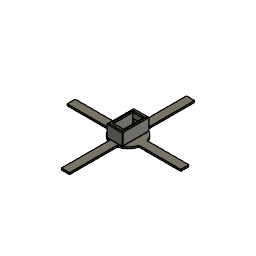
Davinki Base (Autodesk Fusion 360 design; units mm, degrees)
part number: 2026-08-29-10-07-06-773
Autodesk Fusion 360 part; units mm, degrees
note: some values were not read from the file. Set by a fixed rule: which sketch regions a step uses.
sketch "Sketch1" plane through (0, 0, 0) normal (0, 1, 0) x (1, 0, 0)
  line L0 (0, 0) -> (12.25, 0)
  line L1 (12.25, 0) -> (12.25, 23.5)
  line L2 (0, 0) -> (0, 23.5)
  line L3 (0, 23.5) -> (12.25, 23.5)
  line L4 (-3.4056, 0) -> (-3.4056, 27)
  line L5 (-3.4056, 27) -> (15.0988, 27)
  line L6 (15.0988, 27) -> (15.0988, -3.5)
  line L7 (15.0988, -3.5) -> (-3.4056, -3.5)
  line L8 (-3.4056, -3.5) -> (-3.4056, 27)
  line L9 (-3.4056, 27) -> (-3.4056, 28)
  line L10 (-3.4056, 28) -> (15.0988, 28)
  line L11 (15.0988, 28) -> (15.0988, 27)
  line L12 (-3.4056, -3.5) -> (-3.4056, -4.5)
  line L13 (-3.4056, -4.5) -> (15.1, -4.5)
  line L14 (15.1, -4.5) -> (15.0988, -3.5)
  line L15 (0, 23.5) -> (0, 0.25)
  line L16 (5.8472, -4.5) -> (5.8472, -29.5)
  line L17 (5.8472, -29.5) -> (10.8472, -29.5)
  line L18 (10.8472, -29.5) -> (0.8472, -29.5)
  line L19 (0.8472, -29.5) -> (0.8472, -4.5)
  line L20 (10.8472, -29.5) -> (10.8472, -4.5)
  line L21 (5.8466, 28) -> (5.8466, 53)
  line L22 (5.8466, 53) -> (10.8466, 53)
  line L23 (10.8466, 53) -> (0.8466, 53)
  line L24 (0.8466, 53) -> (0.8466, 28)
  line L25 (10.8466, 53) -> (10.8466, 28)
  line L26 (12.25, 11.75) -> (-3.4056, 11.75)
  line L27 (-3.4056, 11.75) -> (-28.4056, 11.75)
  line L28 (-28.4056, 11.75) -> (-28.4056, 6.75)
  line L29 (-28.4056, 6.75) -> (-28.4056, 16.75)
  line L30 (-28.4056, 16.75) -> (-3.4056, 16.7633)
  line L31 (-28.4056, 6.75) -> (-3.4056, 6.75)
  line L32 (15.0988, 11.75) -> (40.0988, 11.75)
  line L33 (40.0988, 11.75) -> (40.0988, 6.75)
  line L34 (40.0988, 6.75) -> (40.0988, 16.75)
  line L35 (40.0988, 16.75) -> (15.0988, 16.75)
  line L36 (40.0988, 6.75) -> (15.0988, 6.75)
  line L37 (-28.4056, 16.75) -> (-63.4056, 16.75)
  line L38 (-28.4056, 6.75) -> (-63.4056, 6.75)
  line L39 (-63.4056, 6.75) -> (-63.4056, 16.75)
  line L40 (40.0988, 16.75) -> (75.0988, 16.75)
  line L41 (75.0988, 16.75) -> (75.0988, 6.75)
  line L42 (75.0988, 6.75) -> (40.0988, 6.75)
  line L43 (10.8466, 53) -> (10.8466, 88)
  line L44 (0.8466, 53) -> (0.8466, 88)
  line L45 (0.8466, 88) -> (10.8466, 88)
  line L46 (10.8472, -29.5) -> (10.8472, -64.5)
  line L47 (10.8472, -64.5) -> (0.8466, -64.5)
  line L48 (0.8466, -64.5) -> (0.8472, -29.5)
  circle A0 centre (5.9954, 11.75) radius 18.8312
  dimension "d1" = 12.25
  dimension "d2" = 23.5
  dimension "d3" = 23.5
  dimension "d6" = 30.5
  dimension "d7" = 1
  dimension "d8" = 1
  dimension "d16" = 23.25
  dimension "d17" = 25
  dimension "d18" = 5
  dimension "d19" = 10
  dimension "d20" = 25
  dimension "d21" = 5
  dimension "d22" = 10
  dimension "d23" = 25
  dimension "d24" = 5
  dimension "d25" = 10
  dimension "d26" = 25
  dimension "d30" = 25
  dimension "d31" = 5
  dimension "d32" = 10
  dimension "d35" = 35
  dimension "d36" = 35
  dimension "d37" = 35
  dimension "d38" = 35
  dimension "d39" = 35
  dimension "d40" = 35
  constraint coincident L0.start L2.start
  constraint horizontal L0
  constraint perpendicular L0 L1
  constraint perpendicular L0 L2
  constraint horizontal L5
  constraint vertical L6
  constraint horizontal L7
  constraint vertical L8
  constraint perpendicular L5 L9
  constraint perpendicular L6 L10
  constraint perpendicular L5 L11
  constraint perpendicular L7 L12
  constraint perpendicular L8 L13
  constraint perpendicular L0 L15
  constraint midpoint L13 L16.start
  constraint perpendicular L13 L16
  constraint perpendicular L16 L17
  constraint perpendicular L16 L18
  constraint coincident L13 L19.end
  constraint perpendicular L13 L19
  constraint perpendicular L17 L20
  constraint midpoint L10 L21.start
  constraint perpendicular L10 L21
  constraint perpendicular L21 L22
  constraint perpendicular L21 L23
  constraint coincident L10 L24.end
  constraint perpendicular L10 L24
  constraint coincident L10 L25.end
  constraint perpendicular L10 L25
  constraint midpoint L1 L26.start
  constraint midpoint L8 L26.end
  constraint perpendicular L4 L26
  constraint perpendicular L8 L27
  constraint perpendicular L27 L28
  constraint perpendicular L27 L29
  constraint coincident L8 L30.end
  constraint perpendicular L8 L31
  constraint midpoint L6 L32.start
  constraint perpendicular L6 L32
  constraint perpendicular L32 L33
  constraint perpendicular L32 L34
  constraint coincident L6 L35.end
  constraint perpendicular L6 L35
  constraint coincident L6 L36.end
  constraint perpendicular L6 L36
  constraint perpendicular L29 L37
  constraint perpendicular L28 L38
  constraint perpendicular L34 L40
  constraint perpendicular L35 L41
  constraint perpendicular L34 L42
  constraint perpendicular L42 L43
  constraint perpendicular L23 L44
  constraint perpendicular L43 L45
  constraint perpendicular L18 L46
  constraint perpendicular L20 L47
  constraint coincident L26 A0.centre
  measures "d1" distance of L0.start L0.end
  measures "d2" distance of L0.end L1.end
  measures "d3" distance of L0.start L2.end
  measures "d6" distance of L4.end L7.end
  measures "d7" distance of L4.end L9.end
  measures "d8" distance of L7.end L12.end
  measures "d16" distance of L2.end L15.end
  measures "d17" distance of L16.start L16.end
  measures "d18" distance of L16.end L17.end
  measures "d19" distance of L17.end L18.end
  measures "d20" distance of L21.start L21.end
  measures "d21" distance of L21.end L22.end
  measures "d22" distance of L22.end L23.end
  measures "d23" distance of L26.end L27.end
  measures "d24" distance of L27.end L28.end
  measures "d25" distance of L28.end L29.end
  measures "d26" distance of L28.end L31.end
  measures "d30" distance of L32.start L32.end
  measures "d31" distance of L32.end L33.end
  measures "d32" distance of L33.end L34.end
  measures "d35" distance of L29.end L37.end
  measures "d36" distance of L28.end L38.end
  measures "d37" distance of L34.end L40.end
  measures "d38" distance of L22.end L43.end
  measures "d39" distance of L23.end L44.end
  measures "d40" distance of L17.end L46.end
extrude "Extrude1" add sketch "Sketch1" along normal blind 17.3 contours L4 L5 L6 L7 L8 | L7 L12 L13 L14 | L5 L9 L10 L11
sketch "Sketch2" plane through (0, 0, -28) normal (0, 0, -1) x (-1, 0, 0)
  line L0 (-15.0988, 0) -> (3.4056, 0)
  line L1 (3.4056, 0) -> (3.4056, 17.3)
  line L2 (3.4056, 17.3) -> (-15.0988, 17.3)
  line L3 (-15.0988, 17.3) -> (-15.0988, 0)
  line L4 (-11.5, 2) -> (-1.0253, 2)
  line L5 (-1.0253, 2) -> (-1.0253, 5)
  line L6 (-11.5, 5) -> (-11.5, 2)
  line L7 (-11.5, 5) -> (-11.5, 10)
  line L8 (-11.5, 10) -> (-1, 10)
  line L9 (-1, 10) -> (-1.0253, 5)
  dimension "d11" = 3
  constraint horizontal L4
  constraint vertical L5
  constraint vertical L6
  constraint perpendicular L7 L8
  measures "d11" distance of L4.start L6.start
extrude "Extrude2" cut sketch "Sketch2" against normal blind 16 contours L4 L5 L6 L7 L8 L9
fillet "Fillet1" radius 1 1 faces at (3.8981, 17.3, 3)
extrude "Extrude3" add sketch "Sketch1" along normal blind 2 contours L4 L8 L27 L31 A0 | L4 L8 L27 L30 A0 | L27 L28 L29 L31 A0 | L27 L29 L30 A0 | L16 L18 L19 A0 | L13 L16 L19 A0 | L6 L32 L36 A0 | L16 L17 L18 L20 A0 | L13 L16 L20 A0 | L6 L32 L35 A0 | L32 L33 L34 L36 A0 | L10 L21 L24 A0 | L21 L23 L24 A0 | L32 L34 L35 A0 | L10 L21 L25 A0 | L21 L22 L23 L25 A0
extrude "Extrude4" add sketch "Sketch1" along normal blind 2 contours L28 L29 L37 L38 L39 | L17 L18 L46 L47 L48 | L33 L34 L40 L41 L42 | L22 L23 L43 L44 L45
extrude "Extrude5" add sketch "Sketch1" along normal blind 2 contours L4 L8 L12 L13 L19 L31 A0 | L6 L13 L14 L20 L36 A0 | L4 L8 L9 L10 L24 L30 A0 | L6 L10 L11 L25 L35 A0
